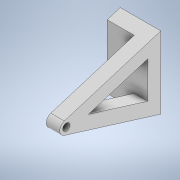
# Autodesk Inventor part: ArrayBracketSupport
Saved by Autodesk Inventor 2022 (Build 260153070, 153G)
## iProperties
Created: 2021-11-28
Part Number: ArrayBracketSupport
Material: Generic
Document SubType Name: Modeling
Designer: elmar
Density: 1 g/cm^3
Appearance: Default
Author: elmar
Autodesk Inventor part; units mm, degrees
ref_plane "YZ Plane" through (0, 0, 0) normal (1, 0, 0) x (0, 1, 0)
ref_plane "XZ Plane" through (0, 0, 0) normal (0, 1, 0) x (-1, 0, 0)
ref_plane "XY Plane" through (0, 0, 0) normal (0, 0, 1) x (1, 0, 0)
sketch "Sketch1" plane through (0, 0, 0) normal (1, 0, 0) x (0, 1, 0)
  circle A0 centre (0, 0) radius 2.9
  line L0 (-2.771, 0.8554) -> (-16, -42)
  line L1 (16, -42) -> (2.771, 0.8554)
  line L2 (43.7128, 0) -> (43.7128, -26)
  line L3 (43.7128, -26) -> (16, -42)
  line L4 (-27.9426, 0) -> (55.6554, 0) projected
  line L5 (8.1395, -36.2) -> (0, -9.832)
  line L6 (0, -9.832) -> (-8.1395, -36.2)
  line L7 (-8.1395, -36.2) -> (8.1395, -36.2)
  line L8 (0, -50.98) -> (0, 11.88) projected
  line L9 (16, -42) -> (-16, -42)
  dimension "d0" = 5.8
  dimension "d1" = 32
  dimension "d2" = 26
  dimension "d4" = 30
  dimension "d19" = 5.8
  dimension "d20" = 32
  constraints: 16 end point, 3 tangent, 2 equal length, 2 point on circle, 2 point on line, 1 centre point, 1 coincident, 1 horizontal, 1 parallel, 1 vertical
  measures "d0" diameter of A0
  measures "d1" distance of L1.start L2.end
  measures "d2" distance of L2.start L2.end
  measures "d4" angle of L4 L3
  measures "d19" distance between parallel lines of L9 L7
  measures "d20" distance of L1.start L0.end
extrude "Extrusion1" add sketch "Sketch1" along normal blind 6 contours L4 L8 A0 | L4 L1 L9 L8 L7 L5 A0 | A0 L8 L4 | A0 L1 L4 | L8 L6 L7 L9 L0 L4 A0 | A0 L4 L8 | L4 A0 L8 | L4 L0 A0
hole "Hole1" at (0, 0, 0) direction (1, 0, 0) diameter 3.2 end through all clearance for "Socket Head Cap Screw" size "M3" standard "Ansi Metric M Profile"
sketch "Sketch3" plane through (0, 0, 0) normal (-1, 0, 0) x (0, 0, 1)
  line L0 (-42, 16) -> (0.8554, 2.771) projected
  line L1 (-42, -16) -> (-42, 16) projected
  line L2 (0.8554, -2.771) -> (-42, -16) projected
  line L3 (-9.832, 0) -> (-36.2, 8.1395) projected
  line L4 (-36.2, -8.1395) -> (-9.832, 0) projected
  line L5 (-36.2, 8.1395) -> (-36.2, -8.1395) projected
  line L6 (-9.832, 0) -> (-36.2, 8.1395) projected
  line L7 (-36.2, 8.1395) -> (-36.2, 14.2096)
  line L8 (-42, 16) -> (0.8554, 2.771) projected
  line L9 (-36.2, 8.1395) -> (-36.2, -8.1395) projected
  line L10 (-36.2, -8.1395) -> (-36.2, -14.2096)
  line L11 (0.8554, -2.771) -> (-42, -16) projected
  arc A0 (0.8554, -2.771) -> (0.8554, 2.771) centre (0, 0) ccw projected
  point P0 (0.1794, -3.245)
  point P1 (0.1794, 3.245)
  point P2 (-36.2, -14.2096)
  point P3 (-36.2, 14.2096)
  constraints: 4 end point, 1 point on line, 1 vertical, 4 other
extrude "Extrusion2" add sketch "Sketch3" along normal blind 12 contours L0 L7 L5 L10 L2 L1
body "Solid1"
